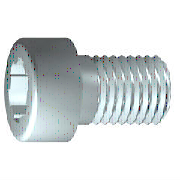
# Autodesk Inventor part: ANSI B18.3 - 1/4-28 UNF - 1.5
Saved by Autodesk Inventor 2016 (Build 200138000, 138)
## iProperties
Created: 2015-02-19
Part Number: ANSI B18.3 - 1/4-28 UNF - 1.5
Material: Steel, Mild
Description: Hexagon Socket Head Cap Screw
Document SubType Name: Modeling
Standard: ANSI B18.3
Designer: steele
Standard Revision: 2003
Standards Organization: ANSI
Language: en-US
Size Designation: 1/4-28 UNF - 1.5
Categories: <MemberInstance><Categories><Category DisplayName="Fasteners" InternalName="e4da775c-781d-43d5-af7c-5136215cf5a6" Mnemonic="FSTN"><Category DisplayName="Bolts" InternalName="536e6df0-f778-49ac-b2f2-25c71d2aa0b2" Mnemonic="SCRW"><CategoryParameter DisplayName="Nominal Diameter Designation" InternalName="03caf894-eafd-4c09-a035-916ac084b87b" Mnemonic="nomdiadesig"/><CategoryParameter DisplayName="Nominal Length" InternalName="238ecbaf-3e6c-45dd-aa95-4068c8e0fd02" Mnemonic="nomlen"/><CategoryParameter DisplayName="Thread Designation" InternalName="586d5e89-370a-4089-914f-0110033585c7" Mnemonic="thrdesign"/><CategoryParameter DisplayName="Thread Series Designation" InternalName="87c5849c-b3a5-4c3e-9c9b-2feecef9be86" Mnemonic="thrserdsgn"/><CategoryParameter DisplayName="Nominal Diameter" InternalName="8bbe3f8e-44cf-40a9-a251-3a6edc8168d6" Mnemonic="nomdia"/><CategoryParameter DisplayName="Thread Type" InternalName="b4bbb7bc-d6aa-4c9f-a9a9-4152b9f6fe49" Mnemonic="thrtype"/><CategoryParameter DisplayName="Thread Pitch" InternalName="bb82302e-82d8-4176-8fc1-c5d7bb17d5ad" Mnemonic="pitch1"/><CategoryParameter DisplayName="Threads per Unit" InternalName="bdc6e7d2-ffd0-4d9c-a173-16b95ebb912d" Mnemonic="thrperunit1"/><CategoryParameter DisplayName="Thread Class" InternalName="ebc0d23b-2cc6-4d2a-b376-d52aae53bab6" Mnemonic="thrclss"/><Category DisplayName="Socket Head" InternalName="55e06bf3-7e58-486c-bbdc-745fcc60664d" Mnemonic="CLSCRW"><CategoryParameter DisplayName="Shank Diameter" InternalName="179dbae3-102f-48bb-85fe-1e3ecd34f7cc" Mnemonic="grpdia"/><CategoryParameter DisplayName="Thread Length" InternalName="3268731d-5f9a-4750-8b01-4a959c46fbf2" Mnemonic="thrlen"/><CategoryParameter DisplayName="Head Diameter" InternalName="46177176-dbdd-4a1b-aefd-4c60c45016af" Mnemonic="headdia"/><CategoryParameter DisplayName="Grip Length" InternalName="52eab69f-422f-4795-9995-175a1b827e67" Mnemonic="grplen"/><CategoryParameter DisplayName="Type" InternalName="59a7e495-7a0c-4a5c-bdfd-c090c5f6e2db" Mnemonic="type"/><CategoryParameter DisplayName="Head Height" InternalName="99c92c4c-4a02-4ebe-9e64-948fb169e19e" Mnemonic="headh"/></Category></Category></Category><Category DisplayName="DataType" InternalName="23b78d0f-2648-40c6-8793-ca6db495c9e8" Mnemonic="DATATYPE"><CategoryParameter DisplayName="DisplayName" InternalName="05415f3d-3907-474b-a020-eb9d644f4cf3" Mnemonic="DISPLAYNAME"/><CategoryParameter DisplayName="Standard" InternalName="0c0a119c-1e12-4c84-803f-101930972f5e" Mnemonic="STANDARD"/><CategoryParameter DisplayName="Description" InternalName="13903e3d-64b1-4950-80da-f627842ea37f" Mnemonic="DESCRIPTION"/><CategoryParameter DisplayName="Designation" InternalName="2675968c-4ce5-49e0-a4f5-552d29089031" Mnemonic="DESIGNATION"/><CategoryParameter DisplayName="Default Row" InternalName="2af9ec52-faaa-4026-b378-f9fa4afca842" Mnemonic="DEFAULTROW"/><CategoryParameter DisplayName="Folder Name" InternalName="3f06958e-8713-4116-9be7-ed6184ecc97b" Mnemonic="FOLDERNAME"/><CategoryParameter DisplayName="Revision Guid" InternalName="45a75005-10b1-4dfc-8d6d-dfe629f0b93c" Mnemonic="REVISIONGUID"/><CategoryParameter DisplayName="FileName" InternalName="8b46a4cc-9585-4fed-90c3-899f57e09a73" Mnemonic="FILENAME"/><CategoryParameter DisplayName="StdsOrg" InternalName="8f5914e1-4693-403f-8ab5-d37768198c9d" Mnemonic="STDSORG"/><CategoryParameter DisplayName="Family Version" InternalName="914462f6-6e19-4b14-ba84-155b9680b1d0" Mnemonic="FAMILYREVISION"/><CategoryParameter DisplayName="Standard Revision" InternalName="91d5a463-65c2-4fde-b823-3b7fea5e8e17" Mnemonic="STANDARDREVISION"/><CategoryParameter DisplayName="Member Revision" InternalName="a65d44b9-392f-4f4f-857b-e4b3d54996fe" Mnemonic="MEMBERREVISION"/><CategoryParameter DisplayName="ClipFormat" InternalName="bc51e27b-3422-4e78-93ef-cec197ddf230" Mnemonic="CLIPFORMAT"/><CategoryParameter DisplayName="Manufacturer" InternalName="cd6c7a72-a28a-4e50-99a9-2c7f4e13e5ad" Mnemonic="MANUFACTURER"/><CategoryParameter DisplayName="InternalName" InternalName="cf1d0246-76d9-4b4a-8305-fa0409afb5c1" Mnemonic="INTERNALNAME"/><CategoryParameter DisplayName="IsMetric" InternalName="e2385c5b-1ea4-4823-96a8-8de651266ec3" Mnemonic="ISMETRIC"/><Category DisplayName="Part" InternalName="c0e0b642-3bcb-4cc8-9e80-f96d35c4afa4" Mnemonic="PART"><CategoryParameter DisplayName="Part Number" InternalName="016b6077-bfbe-49bd-92c9-d8d59c39c941" Mnemonic="PARTNUMBER"/><CategoryParameter DisplayName="Stock Number" InternalName="4dba7c1c-e26c-444e-836c-b08b433409a8" Mnemonic="STOCKNUMBER"/><CategoryParameter DisplayName="Material Key" InternalName="5c9a8adb-dd2b-4535-b97f-0a94a95fe41f" Mnemonic="MATERIALKEY"/><CategoryParameter DisplayName="Material" InternalName="818a152a-d3c3-49ca-80ee-df7d91421b8e" Mnemonic="MATERIAL"/></Category></Category><Category DisplayName="Legacy Map DA" InternalName="924fff40-ddd0-4eff-ad42-30e3774ef79e" Mnemonic="LEGACYMAPDA"><CategoryParameter DisplayName="DACookie" InternalName="316934ee-8fe1-4c7a-9c36-f2d79e1add1a" Mnemonic="DACOOKIE"/></Category><Category DisplayName="LegacyMap" InternalName="cd87c42b-3e48-431e-b5c0-1cbeb14dfe77" Mnemonic="LEGACYMAP"><CategoryParameter DisplayName="unique DA member ID" InternalName="0918ad47-427f-4fed-ae26-24c81c58f590" Mnemonic="DACOOKIE"/><CategoryParameter DisplayName="Merge11 ID" InternalName="0ee8fb18-e2ed-4f39-96f6-1f4b5f50aa71" Mnemonic="MERGE11"/><CategoryParameter DisplayName="unique CC member ID" InternalName="5193edd4-b2b0-4ab4-9d54-de900eee34e0" Mnemonic="CCCOOKIE"/><CategoryParameter DisplayName="Split ID" InternalName="72b5c83c-be7f-45c4-ae51-9160ea6deb26" Mnemonic="SPLIT"/><CategoryParameter DisplayName="MemberID" InternalName="8e5e0294-fc51-4c8f-b3d7-003dc5ed94f6" Mnemonic="MEMBERID"/><CategoryParameter DisplayName="CatalogName" InternalName="d99d1e27-aa94-4de2-af4c-c348882a6f4f" Mnemonic="CATALOGNAME"/><CategoryParameter DisplayName="FamilyNumber" InternalName="e705e1f4-09cb-413e-91f9-551b4188271e" Mnemonic="FAMILYNUMBER"/></Category></Categories><FamilyTemplate Id="sis145"><FamilyTemplateParameters><FamilyTemplateParameter ObjectType="kUserParameterObject" ValueType="xs:double" Id="1" ObjectReferenceKey="GUL"/><FamilyTemplateParameter ObjectType="kUserParameterObject" ValueType="xs:double" Id="2" ObjectReferenceKey="KOH"/><FamilyTemplateParameter ObjectType="kUserParameterObject" ValueType="xs:double" Id="3" ObjectReferenceKey="NLG"/><FamilyTemplateParameter ObjectType="kUserParameterObject" ValueType="xs:double" Id="4" ObjectReferenceKey="KOD"/><FamilyTemplateParameter ObjectType="kUserParameterObject" ValueType="xs:double" Id="5" ObjectReferenceKey="SBR"/><FamilyTemplateParameter ObjectType="kUserParameterObject" ValueType="xs:double" Id="6" ObjectReferenceKey="TOA"/><FamilyTemplateParameter ObjectType="kUserParameterObject" ValueType="xs:double" Id="7" ObjectReferenceKey="GD1"/><FamilyTemplateParameter ObjectType="kUserParameterObject" ValueType="xs:double" Id="8" ObjectReferenceKey="GEL"/><FamilyTemplateParameter ObjectType="kUserParameterObject" ValueType="xs:double" Id="9" ObjectReferenceKey="SW"/><FamilyTemplateParameter ObjectType="kUserParameterObject" ValueType="xs:double" Id="10" ObjectReferenceKey="THREADDIA"/><FamilyTemplateParameter ObjectType="kUserParameterObject" ValueType="xs:double" Id="11" ObjectReferenceKey="SPD"/><FamilyTemplateParameter ObjectType="kUserParameterObject" ValueType="xs:double" Id="12" ObjectReferenceKey="INTI"/><FamilyTemplateParameter ObjectType="kUserParameterObject" ValueType="xs:double" Id="13" ObjectReferenceKey="BDM"/><FamilyTemplateParameter ObjectType="kUserParameterObject" ValueType="xs:double" Id="14" ObjectReferenceKey="ANZ"/><FamilyTemplateParameter ObjectType="kUserParameterObject" ValueType="xs:double" Id="15" ObjectReferenceKey="RR"/><FamilyTemplateParameter ObjectType="kUserParameterObject" ValueType="xs:double" Id="16" ObjectReferenceKey="TPU"/><FamilyTemplateParameter ObjectType="kUserParameterObject" ValueType="xs:double" Id="17" ObjectReferenceKey="PTC"/><FamilyTemplateParameter ObjectType="kUserParameterObject" ValueType="xs:double" Id="18" ObjectReferenceKey="NND"/><FamilyTemplateParameter ObjectType="kUserParameterObject" ValueType="xs:double" Id="19" ObjectReferenceKey="GD"/><FamilyTemplateParameter ObjectType="kUserParameterObject" ValueType="xs:double" Id="20" ObjectReferenceKey="GAL"/><FamilyTemplateParameter ObjectType="kUserParameterObject" ValueType="xs:double" Id="21" ObjectReferenceKey="E0"/><FamilyTemplateParameter ObjectType="kPropertyObject" ValueType="xs:string" Id="100" ObjectReferenceKey="{32853F0F-3444-11d1-9E93-0060B03C1CA6}" SubObjectId="52"/><FamilyTemplateParameter ObjectType="kPropertyObject" ValueType="xs:string" Id="105" ObjectReferenceKey="{32853F0F-3444-11d1-9E93-0060B03C1CA6}" SubObjectId="5"/><FamilyTemplateParameter ObjectType="kPartComponentDefinitionObject" ValueType="xs:string" Id="110" SubObjectId="Material"/><FamilyTemplateParameter ObjectType="kThreadFeatureObject" ValueType="xs:structure" Id="300" ObjectReferenceKey="100200001000000000100000000000008000000000000000" SubObjectId="ThreadInfo"><FamilyTemplateParameter ObjectType="" ValueType="xs:string" Id="301" SubObjectId="ThreadDesignation"/><FamilyTemplateParameter ObjectType="" ValueType="xs:string" Id="302" SubObjectId="ThreadType"/><FamilyTemplateParameter ObjectType="" ValueType="xs:string" Id="303" SubObjectId="ThreadClass"/></FamilyTemplateParameter></FamilyTemplateParameters></FamilyTemplate><CategoryParameterMap><ParamToTemplateMap><ParamToTemplate CategoryParameter="//CategoryParameter[@InternalName='05415f3d-3907-474b-a020-eb9d644f4cf3']" ConstantValue="Spline Socket Head Cap Screw - Inch"/><ParamToTemplate CategoryParameter="//CategoryParameter[@InternalName='cf1d0246-76d9-4b4a-8305-fa0409afb5c1']" ConstantValue="48533e16-23c5-4596-a6af-3b71bb979595"/><ParamToTemplate CategoryParameter="//CategoryParameter[@InternalName='3f06958e-8713-4116-9be7-ed6184ecc97b']" ConstantValue="ANSI B18.3(13)"/><ParamToTemplate CategoryParameter="//CategoryParameter[@InternalName='914462f6-6e19-4b14-ba84-155b9680b1d0']" ConstantValue="10"/><ParamToTemplate CategoryParameter="//CategoryParameter[@InternalName='bc51e27b-3422-4e78-93ef-cec197ddf230']" ConstantValue="CF_INVENTOR.STDPARTS"/><ParamToTemplate CategoryParameter="//CategoryParameter[@InternalName='e2385c5b-1ea4-4823-96a8-8de651266ec3']" ConstantValue="false"/><ParamToTemplate CategoryParameter="//CategoryParameter[@InternalName='13903e3d-64b1-4950-80da-f627842ea37f']" ConstantValue="Hexagon Socket Head Cap Screw"/><ParamToTemplate CategoryParameter="//CategoryParameter[@InternalName='8f5914e1-4693-403f-8ab5-d37768198c9d']" ConstantValue="ANSI"/><ParamToTemplate CategoryParameter="//CategoryParameter[@InternalName='0c0a119c-1e12-4c84-803f-101930972f5e']" ConstantValue="ANSI B18.3"/><ParamToTemplate CategoryParameter="//CategoryParameter[@InternalName='cd6c7a72-a28a-4e50-99a9-2c7f4e13e5ad']" TemplateParameter="104"/><ParamToTemplate CategoryParameter="//CategoryParameter[@InternalName='91d5a463-65c2-4fde-b823-3b7fea5e8e17']" ConstantValue="2003"/><ParamToTemplate CategoryParameter="//CategoryParameter[@InternalName='45a75005-10b1-4dfc-8d6d-dfe629f0b93c']" ConstantValue="c1effc35-3e3a-4cae-b4e4-af135a2ff100"/><ParamToTemplate CategoryParameter="//CategoryParameter[@InternalName='2af9ec52-faaa-4026-b378-f9fa4afca842']" ConstantValue="110"/><ParamToTemplate CategoryParameter="//CategoryParameter[@InternalName='d99d1e27-aa94-4de2-af4c-c348882a6f4f']" ConstantValue="ANSI"/><ParamToTemplate CategoryParameter="//CategoryParameter[@InternalName='8b46a4cc-9585-4fed-90c3-899f57e09a73']" ConstantValue="ANSI B18.3 - 1/4-28 UNF - 1.5(22)"/><ParamToTemplate CategoryParameter="//CategoryParameter[@InternalName='a65d44b9-392f-4f4f-857b-e4b3d54996fe']" ConstantValue="083c0ce7-2809-4e8a-b668-d4339d55600d"/><ParamToTemplate CategoryParameter="//CategoryParameter[@InternalName='52eab69f-422f-4795-9995-175a1b827e67']" ConstantValue="0.5"/><ParamToTemplate CategoryParameter="//CategoryParameter[@InternalName='ebc0d23b-2cc6-4d2a-b376-d52aae53bab6']" ConstantValue="2A"/><ParamToTemplate CategoryParameter="//CategoryParameter[@InternalName='87c5849c-b3a5-4c3e-9c9b-2feecef9be86']" ConstantValue="UNF"/><ParamToTemplate CategoryParameter="//CategoryParameter[@InternalName='03caf894-eafd-4c09-a035-916ac084b87b']" ConstantValue="1/4"/><ParamToTemplate CategoryParameter="//CategoryParameter[@InternalName='b4bbb7bc-d6aa-4c9f-a9a9-4152b9f6fe49']" ConstantValue="ANSI Unified Screw Threads"/><ParamToTemplate CategoryParameter="//CategoryParameter[@InternalName='e705e1f4-09cb-413e-91f9-551b4188271e']" ConstantValue="156"/><ParamToTemplate CategoryParameter="//CategoryParameter[@InternalName='8e5e0294-fc51-4c8f-b3d7-003dc5ed94f6']" ConstantValue="610"/><ParamToTemplate CategoryParameter="//CategoryParameter[@InternalName='316934ee-8fe1-4c7a-9c36-f2d79e1add1a']" ConstantValue="**"/><ParamToTemplate CategoryParameter="//CategoryParameter[@InternalName='179dbae3-102f-48bb-85fe-1e3ecd34f7cc']" TemplateParameter="13"/><ParamToTemplate CategoryParameter="//CategoryParameter[@InternalName='2675968c-4ce5-49e0-a4f5-552d29089031']" TemplateParameter="100"/><ParamToTemplate CategoryParameter="//CategoryParameter[@InternalName='3268731d-5f9a-4750-8b01-4a959c46fbf2']" TemplateParameter="8"/><ParamToTemplate CategoryParameter="//CategoryParameter[@InternalName='46177176-dbdd-4a1b-aefd-4c60c45016af']" TemplateParameter="4"/><ParamToTemplate CategoryParameter="//CategoryParameter[@InternalName='99c92c4c-4a02-4ebe-9e64-948fb169e19e']" TemplateParameter="2"/><ParamToTemplate CategoryParameter="//CategoryParameter[@InternalName='818a152a-d3c3-49ca-80ee-df7d91421b8e']" TemplateParameter="110"/><ParamToTemplate CategoryParameter="//CategoryParameter[@InternalName='238ecbaf-3e6c-45dd-aa95-4068c8e0fd02']" TemplateParameter="3"/><ParamToTemplate CategoryParameter="//CategoryParameter[@InternalName='8bbe3f8e-44cf-40a9-a251-3a6edc8168d6']" TemplateParameter="18"/><ParamToTemplate CategoryParameter="//CategoryParameter[@InternalName='016b6077-bfbe-49bd-92c9-d8d59c39c941']" TemplateParameter="105"/><ParamToTemplate CategoryParameter="//CategoryParameter[@InternalName='bb82302e-82d8-4176-8fc1-c5d7bb17d5ad']" TemplateParameter="17"/><ParamToTemplate CategoryParameter="//CategoryParameter[@InternalName='586d5e89-370a-4089-914f-0110033585c7']" TemplateParameter="301"/><ParamToTemplate CategoryParameter="//CategoryParameter[@InternalName='bdc6e7d2-ffd0-4d9c-a173-16b95ebb912d']" TemplateParameter="16"/></ParamToTemplateMap></CategoryParameterMap></MemberInstance>
Density: 7.85 g/cm^3
Appearance: Semi-Polished
IsCustomPart: 0
Author: steele
Autodesk Inventor part; units mm, degrees
ref_plane "YZ Plane" through (0, 0, 0) normal (1, 0, 0) x (0, 1, 0)
sketch "Sketch1" plane through (0, 0, 0) normal (0, 0, 1) x (1, 0, 0)
  line L0 (-6.35, 0) -> (38.1, 0)
  line L1 (38.1, 0) -> (38.1, 3.175)
  line L2 (38.1, 3.175) -> (0, 3.175)
  line L3 (0, 3.175) -> (0, 4.7625)
  line L4 (-17.3035, 0) -> (47.3339, 0) projected
  line L5 (0, -0.9525) -> (0, 5.715) projected
  line L6 (0, 4.7625) -> (-6.35, 4.7625)
  line L7 (-6.35, 0) -> (-6.35, 4.7625)
  arc A0 (-2.5645, 0) -> (-3.302, 2.7526) centre (-8.0696, 0) ccw
  line L8 (-6.35, 2.7526) -> (-3.302, 2.7526)
  line L9 (12.7, 3.175) -> (0, 3.175) construction
  dimension "d0" = 38.1
  dimension "d1" = 6.35
  dimension "d2" = 6.35
  dimension "d5" = 9.525
  dimension "d13" = 5.5051
  dimension "d14" = 5.5051
  dimension "d15" = 3.048
  constraints: 16 end point, 5 point on line, 3 parallel, 3 perpendicular, 2 collinear, 2 point on circle, 1 centre point, 1 horizontal
  measures "d0" distance between parallel lines of L1 L3
  measures "d1" distance from line of L0.start L3
  measures "d2" diameter of L2 L0
  measures "d5" diameter of L3.end L0
  measures "d13" radius of A0
  measures "d14" diameter of L8 L0
  measures "d15" distance from line of L8.end L7
revolve "Body" add sketch "Sketch1" angle 360 about axis through (-6.35, 0, 0) along (1, 0, 0) contours A0 L8 L7 L6 L3 L5 L0 | L5 L2 L1 L0
ref_plane "IDS_WORKPLANE{1}" through (-6.35, 0, 0) normal (1, 0, 0) x (0, 0, -1)
sketch "Sketch2" plane through (-6.35, 0, 0) normal (1, 0, 0) x (0, 0, -1)
  line L0 (0, -6.6675) -> (0, 6.6675) projected
  line L1 (6.6675, 0) -> (-6.6675, 0) projected
  circle A0 centre (0, 0) radius 4.7625 projected
  line L2 (2.6768, 0.6414) -> (2.2959, 0.6414)
  line L3 (0, 0) -> (2.6768, 0.6414) construction
  line L4 (0, 0) -> (4.0727, 3.8613) construction
  line L5 (0, 0) -> (0.783, 2.6389) construction
  line L6 (0, 0) -> (1.3763, 2.3838) construction
  line L7 (0.783, 2.6389) -> (0.5925, 2.309)
  line L8 (1.8938, 1.9975) -> (1.7034, 1.6676)
  line L9 (0, 0) -> (1.8938, 1.9975) construction
  arc A1 (2.3838, 0) -> (2.2959, 0.6414) centre (0, 0) ccw
  arc A2 (1.7034, 1.6676) -> (0.5925, 2.309) centre (0, 0) ccw
  arc A3 (2.7526, 0) -> (2.6768, 0.6414) centre (0, 0) ccw
  arc A4 (1.8938, 1.9975) -> (0.783, 2.6389) centre (0, 0) ccw
  arc A5 (2.6768, 0.6414) -> (1.6232, 2.223) centre (0, 0) ccw construction
  arc A6 (2.2959, 0.6414) -> (1.7034, 1.6676) centre (0, 0) ccw construction
  line L10 (2.6768, -0.6414) -> (2.2959, -0.6414)
  line L11 (0.783, -2.6389) -> (0.5925, -2.309)
  line L12 (1.8938, -1.9975) -> (1.7034, -1.6676)
  arc A7 (2.2959, -0.6414) -> (2.3838, 0) centre (0, 0) ccw
  arc A8 (0.5925, -2.309) -> (1.7034, -1.6676) centre (0, 0) ccw
  arc A9 (2.6768, -0.6414) -> (2.7526, 0) centre (0, 0) ccw
  arc A10 (0.783, -2.6389) -> (1.8938, -1.9975) centre (0, 0) ccw
  line L13 (-2.6768, 0.6414) -> (-2.2959, 0.6414)
  line L14 (-0.783, 2.6389) -> (-0.5925, 2.309)
  line L15 (-1.8938, 1.9975) -> (-1.7034, 1.6676)
  arc A11 (-2.2959, 0.6414) -> (-2.3838, 0) centre (0, 0) ccw
  arc A12 (-0.5925, 2.309) -> (-1.7034, 1.6676) centre (0, 0) ccw
  arc A13 (-2.6768, 0.6414) -> (-2.7526, 0) centre (0, 0) ccw
  arc A14 (-0.783, 2.6389) -> (-1.8938, 1.9975) centre (0, 0) ccw
  line L16 (-0.783, -2.6389) -> (-0.5925, -2.309)
  arc A15 (-1.7034, -1.6676) -> (-0.5925, -2.309) centre (0, 0) ccw
  line L17 (-1.8938, -1.9975) -> (-1.7034, -1.6676)
  arc A16 (-1.8938, -1.9975) -> (-0.783, -2.6389) centre (0, 0) ccw
  arc A17 (-2.3838, 0) -> (-2.2959, -0.6414) centre (0, 0) ccw
  line L18 (-2.6768, -0.6414) -> (-2.2959, -0.6414)
  arc A18 (-2.7526, 0) -> (-2.6768, -0.6414) centre (0, 0) ccw
  point P0 (1.3763, -2.3838)
  point P1 (-1.3763, 2.3838)
  point P2 (-1.3763, -2.3838)
  dimension "d19" = 0.6413
  dimension "d20" = 1.2827
  dimension "d21" = 33.052
  dimension "d22" = 5.5051
  dimension "d23" = 4.7676
  constraints: 40 point on circle, 34 end point, 26 symmetric about line, 18 centre point, 7 coincident, 2 parallel, 2 point on line, 23 other
  measures "d19" distance between parallel lines of L2 L1
  measures "d20" distance between parallel lines of L7 L8
  measures "d21" angle of L9 L3
  measures "d22" diameter of A5
  measures "d23" diameter of A6
extrude "Slot" add sketch "Sketch2" along normal up to next contours A1 L2 A3 L1 | L1 A9 L10 A7 | A17 L18 A18 L1 | L1 A13 L13 A11 | A4 L8 A2 L7 | L11 A8 L12 A10 | L14 A12 L15 A14 | A16 L17 A15 L16
fillet "Fillet1" radius 0.635 1 edges at (-6.35, -4.7625, 0)
thread "Thread" size "1/4-28 UNF" class "2A" standard "ANSI Unified Screw Threads" length 25.4
chamfer "Chamfer1" distance 0.541 distance2 0.541 1 edges at (38.1, -3.175, 0) measured on face at (38.1, -0.6107, -1.4381)
ref_plane "Work Plane2" through (-3.175, 0, 0) normal (0, 0, -1) x (1, 0, 0)
equation "\"d19\" = 0.5 * SBR"
equation "\"d20\" = SBR"
equation "\"d22\" = 1.1547 * SW"
equation "\"d23\" = SW"
equation "\"d17\" = INTI"
equation "\"d24\" = RR"
equation "\"d6\" = GEL"
equation "\"d9\" = -0.5 * SPD + 0.5 * NND"
equation "\"d10\" = GUL"
equation "\"d0\" = NLG"
equation "\"d1\" = KOH"
equation "\"d2\" = NND"
equation "\"d5\" = KOD"
equation "\"d13\" = 1.1547 * SW"
equation "\"d14\" = 1.1547 * SW"
equation "\"d15\" = INTI"
equation "\"NND\" = 6.35"
equation "\"NLG\" = 38.1"
equation "\"GEL\" = 25.4"
equation "\"KOD\" = 9.525"
equation "\"KOH\" = 6.35"
equation "\"SPD\" = GD1"
equation "\"GUL\" = 0.54102"
equation "\"SBR\" = 1.2827"
equation "\"INTI\" = 3.048"
equation "\"d11\" = -KOH"
equation "\"SW\" = 4.76758"
equation "\"d16\" = 1.1547 * SW"
equation "\"d18\" = SW"
equation "\"RR\" = 0.635"
equation "\"TOA\" = 30deg"
equation "\"GD1\" = 5.26796"
equation "\"THREADDIA\" = 6.35"
equation "\"BDM\" = NND"
equation "\"GD\" = NND"
equation "\"GAL\" = 1.36068"
equation "\"E0\" = 5.55498"
body "Solid1"
